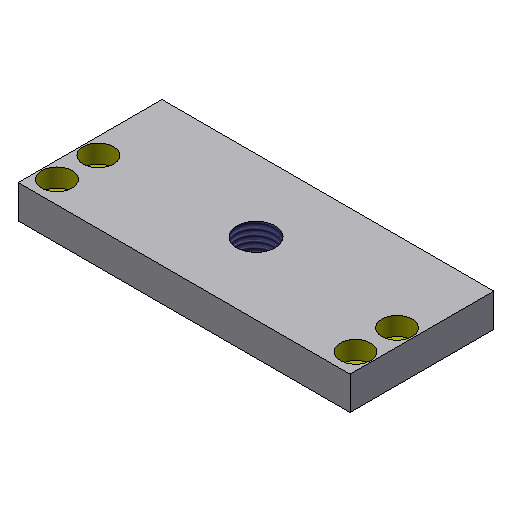
# Autodesk Inventor part: TL20240701-10110CV-004
Saved by Autodesk Inventor 2022.5 (Build 265521000, 521)
## iProperties
Category: DRIVE UNIT ASSY
Company: 현대 트랜시스(대유)
Created: 2023-05-17
Part Number: TL20240701-10110CV-004
Checked By: 김형민
Engr Approved By: 김시현
User Status: 4 x18
Material: SS400
Description: 0
Document SubType Name: Modeling
Mfg Approved By: 호상태
Designer: 길창현
Stock Number: 004
Density: 7.85 g/cm^3
Appearance: Painting-RAL7035
Project: SW PJT
DETAIL: Coveryor Assembly
M/C TITLE: CJ 제일제당 협동로봇 포장시스탬 PILOT 장비
PARTS NAME: Bracket
SPECIFICATION: TA20221101-CV200000-015
DocNumber: 221118_Standard_v1
Folder: .\
VDS_Category: 엔지니어링
Detail Description: Processed products
Title: BLOCK
Subject: SW차종 시트조립라인
Author: 길창현
Revision Number: A
Autodesk Inventor part; units mm, degrees
ref_plane "YZ Plane" through (0, 0, 0) normal (1, 0, 0) x (0, 1, 0)
ref_plane "XZ Plane" through (0, 0, 0) normal (0, 1, 0) x (-1, 0, 0)
ref_plane "XY Plane" through (0, 0, 0) normal (0, 0, 1) x (1, 0, 0)
sketch "스케치9" plane through (0, 0, 0) normal (0, 0, 1) x (1, 0, 0)
  line L0 (-60, 26) -> (60, 26)
  line L1 (60, 26) -> (60, -26)
  line L2 (60, -26) -> (-60, -26)
  line L3 (-60, -26) -> (-60, 26)
  line L4 (-60, 26) -> (60, -26) construction
  line L5 (60, 26) -> (-60, -26) construction
  point P0 (0, 0)
  dimension "d40" = 120
  dimension "d41" = 52
  constraints: 12 end point, 2 midpoint, 2 parallel, 1 horizontal, 1 perpendicular
  measures "d40" distance of L1.end L2.end
  measures "d41" distance of L0.end L1.end
extrude "돌출4" add sketch "스케치9" along normal mid plane 12
sketch "스케치10" plane through (0, 0, 6) normal (0, 0, 1) x (1, 0, 0)
  point P0 (0, 0)
  point P1 (0, 0)
  constraints: 1 coincident
hole "구멍3" at (0, 0, 6) direction (0, 0, -1) diameter 13.835 end through all thread size "M16x2" class "6H" standard "ISO Metric profile"
sketch "스케치11" plane through (0, 0, 6) normal (0, 0, 1) x (1, 0, 0)
  line L0 (54, -3) -> (54, -18)
  line L1 (-54, -3) -> (-54, -18)
  line L2 (60, -26) -> (60, 26) projected
  line L3 (-60, 26) -> (-60, -26) projected
  line L4 (-60, -26) -> (60, -26) projected
  point P0 (0, 0)
  point P1 (-60, 0)
  point P2 (60, 0)
  dimension "d51" = 6
  dimension "d52" = 6
  dimension "d53" = 8
  dimension "d54" = 15
  constraints: 4 end point, 2 midpoint, 2 vertical, 1 horizontal alignment, 1 parallel
  measures "d51" distance between parallel lines of L2 L0
  measures "d52" distance between parallel lines of L3 L1
  measures "d53" distance from line of L4 L0.end
  measures "d54" distance of L0.start L0.end
hole "구멍4" at (-54, -3, 6) at (-54, -18, 6) at (54, -18, 6) at (54, -3, 6) direction (0, 0, -1) diameter 6.6 end through all counterbore diameter 11 counterbore depth 6.6 clearance for "Hex Head Cap Screw DIN EN 24017" size "M6" standard "DIN"
sketch "스케치12" plane through (-60, 26, 6) normal (0, 1, 0) x (1, 0, 0)
  line L0 (0, 12) -> (0, 0) projected
  line L1 (120, 12) -> (120, 0) projected
  point P0 (60, 6)
  point P1 (20, 6)
  point P2 (35, 6)
  point P3 (85, 6)
  point P4 (100, 6)
  point P5 (0, 6)
  dimension "d62" = 120
  dimension "d63" = 20
  dimension "d64" = 15
  dimension "d76" = 20
  dimension "d77" = 15
  constraints: 5 horizontal alignment, 1 midpoint
  measures "d62" distance between parallel lines of L0 L1
  measures "d63" distance from line of point (20, 6) L0
  measures "d64" distance of point (35, 6) point (20, 6)
  measures "d76" distance from line of L1 point (100, 6)
  measures "d77" distance of point (85, 6) point (100, 6)
hole "구멍5" at (-40, 26, 0) at (-25, 26, 0) at (25, 26, 0) at (40, 26, 0) direction (0, -1, 0) diameter 4.917 depth 17.1 tip angle 118 thread size "M6x1" class "6H" standard "ISO Metric profile"
